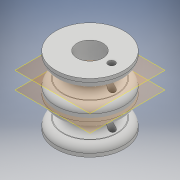
# Autodesk Inventor part: MotorPully
Saved by Autodesk Inventor 2017 (Build 210142000, 142)
## iProperties
Created: 2017-02-15
Part Number: MotorPully
Material: Generic
Document SubType Name: Modeling
Designer: aribu
Density: 1 g/cm^3
Appearance: Default
Author: aribu
Autodesk Inventor part; units mm, degrees
ref_plane "YZ Plane" through (0, 0, 0) normal (1, 0, 0) x (0, 1, 0)
ref_plane "XZ Plane" through (0, 0, 0) normal (0, 1, 0) x (-1, 0, 0)
ref_plane "XY Plane" through (0, 0, 0) normal (0, 0, 1) x (1, 0, 0)
sketch "Sketch1" plane through (0, 0, 0) normal (0, 0, 1) x (1, 0, 0)
  circle A0 centre (0, 0) radius 5
  dimension "d0" = 10
  constraints: 1 centre point, 1 coincident
  measures "d0" diameter of A0
extrude "Extrusion1" add sketch "Sketch1" along normal blind 10
ref_plane "Work Plane2" through (0, 0, 7.5) normal (0, 0, 1) x (1, 0, 0)
ref_plane "Work Plane1" through (0, 0, 5) normal (0, 0, 1) x (1, 0, 0)
sketch "Sketch2" plane through (0, 0, 7.5) normal (0, 0, 1) x (1, 0, 0)
  circle A0 centre (0, 0) radius 5
  circle A1 centre (0, 0) radius 2.9
  dimension "d3" = 5.8
  dimension "d4" = 10
  constraints: 2 centre point, 2 coincident
  measures "d3" diameter of A1
  measures "d4" diameter of A0
extrude "Extrusion2" cut sketch "Sketch2" along normal mid plane 2
mirror "Mirror1" about plane through (0, 0, 5) normal (0, 0, 1) of "Extrusion2"
fillet "Fillet1" radius 1 4 edges at (-5, 0, 6.5) (-5, 0, 8.5) (-5, 0, 3.5) (-5, 0, 1.5)
fillet "Fillet2" radius 1 4 edges at (-2.9, 0, 6.5) (-2.9, 0, 8.5) (-2.9, 0, 3.5) (-2.9, 0, 1.5)
sketch "Sketch3" plane through (0, 0, 0) normal (0, 0, -1) x (-1, 0, 0)
  point P0 (0, 0)
sketch "Sketch4" plane through (0, 0, 0) normal (0, 0, -1) x (-1, 0, 0)
  circle A0 centre (0, 0) radius 1.9
  dimension "d11" = 3.8
  constraints: 1 centre point, 1 coincident
  measures "d11" diameter of A0
extrude "Extrusion3" cut sketch "Sketch4" against normal blind 10
sketch "Sketch5" plane through (0, 0, 0) normal (0, 0, -1) x (-1, 0, 0)
  circle A0 centre (0, 0) radius 3.375 projected
  circle A1 centre (-3.1668, 0) radius 0.5
  dimension "d16" = 1
  constraints: 1 centre point
  measures "d16" diameter of A1
extrude "Extrusion4" cut sketch "Sketch5" against normal blind 10 contours A1 A0 | A0 A1 picked at (-3.1365, 0) picked at (-3.4698, 0)
body "Solid1"
